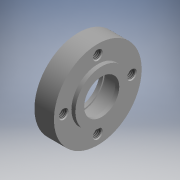
# Autodesk Inventor part: BARR608ZZ_b
Saved by Autodesk Inventor 2017.3 (Build 213256000, 256)
## iProperties
Part Number: BARR608ZZ_b
Material: Generic
Catalog Web Link: www.cadenas.de
Description: BGRRB, BGRR, BARR, SBARR, SBGRR_body-Bearings with Housing - Standard with Pilots - Round
Vendor: MISUMI
Document SubType Name: Modeling
Designer: partserver
Manufacturer: MISUMI
Mass: 11.4818 g
Surface Area: 57.7363 cm^2
Volume: 11.4818 cm^3
Density: 1 g/cm^3
Appearance: PSOLRGB-192-192-192
Category: PARTsolutions
Company: MISUMI
Title: BARR608ZZ
Author: Cadenas PARTsolutions
Comments: Bearings with Housing - Standard with Pilots - Round
PSOL_IDENT_0: {$CADENAS_DATA\23d-libs\misumi\metric\12_bearing_holders\bgrrb\bgrrb_housing.prj},213 {VTYP=3D},{NB=
PSOL_IDENT_1: BARR608ZZ_b},{LINA=BARR608ZZ},{NN=BGRRB, BGRR, BARR, SBARR, SBGRR_body},{DATE=30.03.2018 01:48:28},{
PSOL_IDENT_2: GEOMDATE=18.08.2015 01:55:07},{VERSION=},{LINEID=70},{WBVAR=MATB,MATH,ST,SEALT,ALT1},{WBNUMERIC=}  {
PSOL_IDENT_3: NB=BARR608ZZ_b},{LINA=BARR608ZZ},{KT=DUMMY},{PN=BARR608ZZ},{TYPE=BARR},{MATB=},{MATBALG=  '', 'Steel'
PSOL_IDENT_4: , 'S', 'Stainless Steel'  },{MATH=A2000},{ST=CA},{ST1=  'CA','Clear Anodize'  },{AC=304 Stainless St
PSOL_IDENT_5: eel},{BN=608},{BN2=608.000},{SEALT=ZZ},{MS=0.000},{MS2=0.000},{DD=8},{D=22},{D3=23.500},{TR=1.15},{B=
PSOL_IDENT_6: 7},{H=45},{T=12},{T1=10},{S=2},{LL1=2},{DDHH=18},{D1G7=27},{PCD=35},{F=0},{D2=M 5 (4.3)},{DD1=8.0},{
PSOL_IDENT_7: H1=4.4},{MATH1=  'S45CE','1045 Carbon Steel Equivalent','A2000','2000 Aluminum Alloy'    },{D2MIN=4.
PSOL_IDENT_8: 300},{D2MAX=5.000},{NR=},{SEALTALG= 'ZZ','ZZ(Double Shielded)','VV','VV(Non-Contact Sealed Rubber Se
PSOL_IDENT_9: al)','DD','DD(Contact Sealed Rubber Seal)' },{BNHALG=1},{ALT1=},{ALT1ALG= '', 'Bearing and Retaining
PSOL_IDENT_10: Ring Assembled', '-NA'  , 'with NA (Bearing and Retaining Ring not Assembled)'}
NB: BARR608ZZ_b
NN: BGRRB, BGRR, BARR, SBARR, SBGRR_body
NT: Bearings with Housing - Standard with Pilots - Round
NBSYN: $PN._b
LINA: BARR608ZZ
CATALOG: Misumi
PN: BARR608ZZ
MATB: Steel
MATH: 2000 Aluminum Alloy
ST: Clear Anodize
AC: 304 Stainless Steel
BN: 608
SEALT: ZZ(Double Shielded)
DD: 8
D: 22
B: 7
H: 45
T: 12
T1: 10
S: 2
LL1: 2
DDHH: 18
D1G7: 27
PCD: 35
F: 0
D2: M 5 (4.3)
DD1: 8
H1: 4.4
ALT1: Bearing and Retaining Ring Assembled
SUPPLIER: MISUMI
ARTICLENO: BARR608ZZ_b
BOMINFO: BARR608ZZ
CREATOR: CADENAS GmbH
Autodesk Inventor part; units mm, degrees
sketch "Sketch_1" plane through (0, 0, 0) normal (1, 0, 0) x (0, 1, 0)
  circle A0 centre (0, 0) radius 22.5
  constraints: 1 centre point
extrude "Extrusion1" add sketch "Sketch_1" along normal blind 12
sketch "Sketch_2" plane through (0, 0, 0) normal (0, 0, 1) x (1, 0, 0)
  line L0 (12, 0) -> (0, 0)
  line L1 (0, 0) -> (0, 9)
  line L2 (0, 9) -> (2, 9)
  line L3 (2, 9) -> (2, 11)
  line L4 (2, 11) -> (9, 11)
  line L5 (9, 11) -> (9, 11.75)
  line L6 (9, 11.75) -> (10.15, 11.75)
  line L7 (10.15, 11.75) -> (10.15, 11)
  line L8 (10.15, 11) -> (12, 11)
  line L9 (12, 11) -> (12, 0)
  line L10 (12, 0) -> (0, 0)
  constraints: 22 end point
revolve "Revolution1" cut sketch "Sketch_2" angle 360 about axis through (12, 0, 0) along (1, 0, 0)
sketch "Sketch_9" plane through (0, 0, 0) normal (0, 0, 1) x (1, 0, 0)
  line L0 (12, 17.5) -> (2, 17.5)
  line L1 (2, 17.5) -> (2, 20)
  line L2 (2, 20) -> (2.433, 19.567)
  line L3 (2.433, 19.567) -> (7.167, 19.567)
  line L4 (7.167, 19.567) -> (7.6, 20)
  line L5 (7.6, 20) -> (7.6, 21.5)
  line L6 (7.6, 21.5) -> (12, 21.5)
  line L7 (12, 21.5) -> (12, 17.5)
  line L8 (12, 17.5) -> (2, 17.5)
  constraints: 18 end point
revolve "Revolution2" cut sketch "Sketch_9" angle 360 about axis through (12, 17.5, 0) along (1, 0, 0)
thread "Thread1" size "M5x0.8" class "6H" standard "ISO Metric profile" full length
sketch "Sketch_4" plane through (0, 0, 0) normal (1, 0, 0) x (0, 1, 0)
  circle A0 centre (0, 0) radius 46
  circle A1 centre (0, 0) radius 13.5
  constraints: 2 centre point
extrude "Extrusion2" cut sketch "Sketch_4" along normal blind 2
pattern_linear "Rectangular Pattern1" count 2 spacing 24.7487 along (0, -0.7071, 0.7071) count 2 spacing 24.7487 along (0, -0.7071, -0.7071) of "Revolution2"
ref_plane "bgrrb_to_rring_XY" through (9, 0, 0) normal (1, 0, 0) x (0, 0, -1)
ref_plane "bgrrb_to_rring_YZ" through (9, 0, 0) normal (0, 0, -1) x (0, 1, 0)
ref_plane "bgrrb_to_rring_ZX" through (9, 0, 0) normal (0, 1, 0) x (1, 0, 0)
ref_plane "housing_to_dummy_XY" through (0, 0, 0) normal (0, 0, 1) x (1, 0, 0)
ref_plane "housing_to_dummy_YZ" through (0, 0, 0) normal (1, 0, 0) x (0, 1, 0)
ref_plane "housing_to_dummy_ZX" through (0, 0, 0) normal (0, 1, 0) x (0, 0, 1)
ref_plane "to_bearings_1_XY" through (2, 0, 0) normal (1, 0, 0) x (0, 0, -1)
ref_plane "to_bearings_1_YZ" through (2, 0, 0) normal (0, 0, -1) x (0, 1, 0)
ref_plane "to_bearings_1_ZX" through (2, 0, 0) normal (0, 1, 0) x (1, 0, 0)
body "Solid1"
